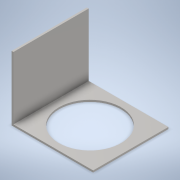
# Autodesk Inventor part: ammonia filter bracket
Saved by Autodesk Inventor 2020 (Build 240168000, 168)
## iProperties
Created: 2020-08-10
Part Number: ammonia filter bracket
Material: Generic
Document SubType Name: Modeling
Designer: Abbas
Density: 1 g/cm^3
Appearance: Default
Author: Abbas
Autodesk Inventor part; units mm, degrees
ref_plane "YZ Plane" through (0, 0, 0) normal (1, 0, 0) x (0, 1, 0)
ref_plane "XZ Plane" through (0, 0, 0) normal (0, 1, 0) x (-1, 0, 0)
ref_plane "XY Plane" through (0, 0, 0) normal (0, 0, 1) x (1, 0, 0)
sketch "Sketch1" plane through (0, 0, 0) normal (0, 1, 0) x (-1, 0, 0)
  circle A0 centre (0, 0) radius 49.5
  line L0 (65, 60) -> (-65, 60)
  line L1 (-65, 60) -> (-65, -60)
  line L2 (-65, -60) -> (65, -60)
  line L3 (65, -60) -> (65, 60)
  line L4 (65, 60) -> (-65, -60) construction
  line L5 (-65, 60) -> (65, -60) construction
  dimension "d0" = 99
  dimension "d1" = 130
  dimension "d2" = 120
  constraints: 12 end point, 2 midpoint, 2 parallel, 1 centre point, 1 coincident, 1 horizontal, 1 perpendicular
  measures "d0" diameter of A0
  measures "d1" distance of L2.end L1.end
  measures "d2" distance of L1.end L0.end
extrude "Extrusion1" add sketch "Sketch1" along normal blind 3
sketch "Sketch2" plane through (0, 3, 0) normal (0, 1, 0) x (1, 0, 0)
  line L0 (-65, -60) -> (-62, -60)
  line L1 (-62, -60) -> (-62, 60)
  line L2 (-62, 60) -> (-65, 60)
  line L3 (-65, 60) -> (-65, -60)
  line L4 (-65, -60) -> (-62, 60) construction
  line L5 (-62, -60) -> (-65, 60) construction
  line L6 (-65, 60) -> (-65, -60) projected
  point P0 (0, 0)
  point P1 (-63.5, 0)
  point P2 (-65, 0)
  dimension "d5" = 3
  dimension "d6" = 120
  constraints: 12 end point, 4 midpoint, 2 parallel, 1 horizontal, 1 perpendicular
  measures "d5" distance of L2.end L1.end
  measures "d6" distance of L1.end L0.end
extrude "Extrusion2" add sketch "Sketch2" along normal blind 100
body "Solid1"
